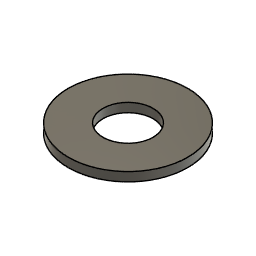
seat mount aft v4 (Autodesk Fusion 360 archive; units mm, degrees)
design "M8x20 washer"
Autodesk Fusion 360 part; units mm, degrees
sketch "Sketch1" plane through (0, 0, 0) normal (0, 1, 0) x (1, 0, 0)
  circle A0 centre (0, 0) radius 4.2
  circle A1 centre (0, 0) radius 10
  dimension "d1" = 8.4
  dimension "d2" = 20
  constraint coincident A0.centre A1.centre
  constraint concentric A0 A1
  measures "d1" diameter of A0
  measures "d2" diameter of A1
extrude "Extrude1" add sketch "Sketch1" along normal blind 1.5 makes body 1
copy_body "Body->Comp1" bodies 1 removing the originals makes body 2 in component "M8x20 washer"
component "M8x20 washer" placed x (1, 0, 0) y (0, 1, 0) z (0, 0, 1) at (0, 0, 0)
named bodies: "M8x20 washer"
